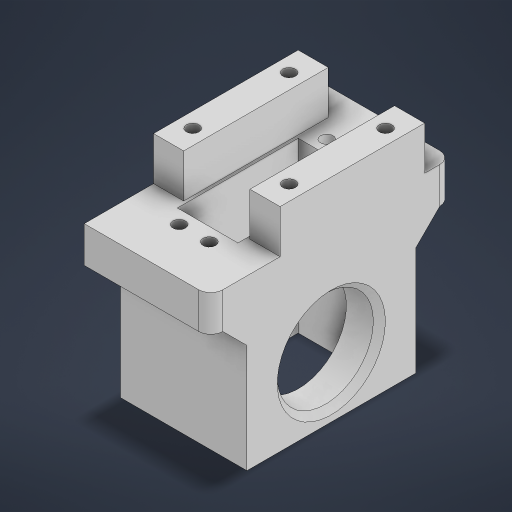
# Autodesk Inventor part: VerticalAxisServoMount
Saved by Autodesk Inventor 2024 (Build 280153000, 153)
## iProperties
Created: 2024-01-29
Part Number: VerticalAxisServoMount
Material: Generic
Document SubType Name: Modeling
Designer: avsar
Density: 1 g/cm^3
Appearance: Default
Author: avsar
Autodesk Inventor part; units mm, degrees
ref_plane "YZ Plane" through (0, 0, 0) normal (1, 0, 0) x (0, 1, 0)
ref_plane "XZ Plane" through (0, 0, 0) normal (0, 1, 0) x (-1, 0, 0)
ref_plane "XY Plane" through (0, 0, 0) normal (0, 0, 1) x (1, 0, 0)
sketch "Sketch1" plane through (0, 0, 0) normal (1, 0, 0) x (0, 1, 0)
  circle A0 centre (0, 0) radius 15.95
  dimension "d0" = 31.9
  constraints: 1 centre point, 1 coincident
  measures "d0" diameter of A0
extrude "Extrusion1" add sketch "Sketch1" along normal blind 8
sketch "Sketch2" plane through (8, 0, 0) normal (1, 0, 0) x (0, 0, -1)
  line L0 (-28, -20) -> (28, -20)
  line L1 (28, -20) -> (28, 36)
  line L2 (28, 36) -> (-28, 36)
  line L3 (-28, 36) -> (-28, -20)
  line L4 (-28, -20) -> (28, 36) construction
  line L5 (28, -20) -> (-28, 36) construction
  point P0 (0, 0)
  point P1 (0, 8)
  point P2 (0, 8)
  dimension "d3" = 56
  dimension "d4" = 56
  dimension "d46" = 8
  constraints: 12 end point, 2 midpoint, 2 parallel, 1 horizontal, 1 perpendicular, 1 vertical alignment
  measures "d3" distance of L1.end L0.end
  measures "d4" distance of L1.end L2.end
  measures "d46" distance of point (0, 0) point (0, 8)
extrude "Extrusion2" add sketch "Sketch2" along normal blind 42
sketch "Sketch3" plane through (8, 36, 28) normal (0, 1, 0) x (1, 0, 0)
  line L0 (0, 56) -> (42, 56) projected
  line L1 (21, 56) -> (21, 0) construction
  line L2 (0, 0) -> (42, 0) projected
  line L3 (10.95, 7.95) -> (31.05, 7.95)
  line L4 (31.05, 7.95) -> (31.05, 48.05)
  line L5 (31.05, 48.05) -> (10.95, 48.05)
  line L6 (10.95, 48.05) -> (10.95, 7.95)
  line L7 (10.95, 7.95) -> (31.05, 48.05) construction
  line L8 (31.05, 7.95) -> (10.95, 48.05) construction
  point P0 (-8, 28)
  point P1 (21, 28)
  dimension "d7" = 20.1
  dimension "d8" = 40.1
  constraints: 14 end point, 5 midpoint, 2 parallel, 1 horizontal, 1 perpendicular
  measures "d7" distance of L5.end L4.end
  measures "d8" distance of L4.end L3.end
extrude "Extrusion3" cut sketch "Sketch3" against normal through all
sketch "Sketch4" plane through (50, 0, 0) normal (1, 0, 0) x (0, 0, -1)
  circle A0 centre (0, 0) radius 15.95 projected
extrude "Extrusion4" cut sketch "Sketch4" against normal up to surface (10.95 mm away)
sketch "Sketch5" plane through (18.95, 36, 20.05) normal (1, 0, 0) x (0, 0, -1)
  circle A0 centre (20.05, -36) radius 15.95 construction
  circle A1 centre (12.05, -28) radius 2.1
  circle A2 centre (12.05, -44) radius 2.1
  circle A3 centre (28.05, -44) radius 2.1
  circle A4 centre (28.05, -28) radius 2.1
  dimension "d13" = 4.2
  dimension "d14" = 8
  dimension "d15" = 8
  dimension "d18" = 360
  constraints: 4 centre point, 9 other
  measures "d13" diameter of A1
  measures "d14" horizontal distance of A1.centre point (20.05, -36)
  measures "d15" horizontal distance of point (20.05, -36) A1.centre
extrude "Extrusion5" cut sketch "Sketch5" against normal through all
sketch "Sketch6" plane through (8, 36, 28) normal (0, 1, 0) x (1, 0, 0)
  line L0 (31.05, 48.05) -> (10.95, 48.05) construction
  line L1 (21, 48.05) -> (21, 7.95) construction
  line L2 (10.95, 7.95) -> (31.05, 7.95) construction
  line L3 (0, 0) -> (42, 0) projected
  line L4 (0, 0) -> (42, 0)
  line L5 (42, 0) -> (42, -12)
  line L6 (42, -12) -> (0, -12)
  line L7 (0, -12) -> (0, 0)
  line L8 (10.95, 7.95) -> (10.95, 48.05) construction
  line L9 (10.95, 28) -> (31.05, 28) construction
  line L10 (31.05, 12.05) -> (31.05, 43.95) construction
  line L11 (0, 56) -> (42, 56)
  line L12 (0, 56) -> (42, 56)
  line L13 (42, 56) -> (42, 68)
  line L14 (42, 68) -> (0, 68)
  line L15 (0, 68) -> (0, 56)
  point P0 (-8, 28)
  point P1 (21, 28)
  dimension "d25" = 12
  constraints: 22 end point, 5 midpoint, 5 symmetric about line, 2 parallel, 1 coincident, 1 horizontal, 1 perpendicular
  measures "d25" distance of L4.end L5.end
extrude "Extrusion6" add sketch "Sketch6" against normal blind 12
sketch "Sketch8" plane through (8, 36, 40) normal (0, 1, 0) x (1, 0, 0)
  line L0 (10.95, 19.95) -> (31.05, 19.95) construction
  line L1 (21, 19.95) -> (21, 60.05) construction
  line L2 (31.05, 60.05) -> (10.95, 60.05) construction
  circle A0 centre (26, 15.5) radius 2.1
  line L3 (31.05, 19.95) -> (10.95, 19.95) projected
  line L4 (10.95, 19.95) -> (10.95, 60.05) construction
  line L5 (10.95, 40) -> (31.05, 40) construction
  line L6 (31.05, 24.05) -> (31.05, 55.95) construction
  circle A1 centre (16, 15.5) radius 2.1
  circle A2 centre (26, 64.5) radius 2.1
  circle A3 centre (16, 64.5) radius 2.1
  point P0 (-8, 40)
  point P1 (21, 19.95)
  point P2 (21, 40)
  dimension "d31" = 4.2
  dimension "d32" = 5
  dimension "d33" = 24.5
  constraints: 6 midpoint, 4 centre point, 4 end point, 3 symmetric about line, 3 other
  measures "d31" diameter of A0
  measures "d32" horizontal distance of point (21, 19.95) A0.centre
  measures "d33" vertical distance of point (21, 40) A0.centre
extrude "Extrusion8" cut sketch "Sketch8" against normal up to surface (12 mm away)
fillet "Fillet2" radius 4 2 edges at (50, 30, 40) (50, 30, -40)
chamfer "Chamfer1" distance 2 angle 45 1 edges at (50, 0, 15.95)
chamfer "Chamfer2" distance 8 angle 45 2 edges at (29, 24, 28) (29, 24, -28)
sketch "Sketch10" plane through (8, 36, 40) normal (0, 1, 0) x (1, 0, 0)
  line L0 (31.05, 60.05) -> (10.95, 60.05) construction
  line L1 (21, 60.05) -> (21, 19.95) construction
  line L2 (31.05, 19.95) -> (10.95, 19.95) construction
  circle A0 centre (5, 31) radius 2.1
  circle A1 centre (5, 63) radius 2.1
  circle A2 centre (37, 31) radius 2.1
  circle A3 centre (37, 63) radius 2.1
  line L3 (0, 80) -> (0, 0) construction
  line L4 (0, 71) -> (10, 71)
  line L5 (10, 71) -> (10, 23)
  line L6 (10, 23) -> (0, 23)
  line L7 (0, 23) -> (0, 71)
  line L8 (5, 63) -> (5, 31) construction
  line L9 (42, 71) -> (32, 71)
  line L10 (32, 71) -> (32, 23)
  line L11 (32, 23) -> (42, 23)
  line L12 (42, 23) -> (42, 71)
  point P0 (-8, 40)
  point P1 (21, 40)
  point P2 (10, 47)
  point P3 (5, 47)
  dimension "d58" = 4.2
  dimension "d59" = 9
  dimension "d60" = 16
  dimension "d61" = 4.2
  dimension "d62" = 32
  dimension "d63" = 48
  dimension "d64" = 10
  constraints: 20 end point, 6 symmetric about line, 5 midpoint, 4 centre point, 2 parallel, 1 horizontal, 1 horizontal alignment, 1 perpendicular, 1 point on line, 1 vertical, 1 vertical alignment, 2 other
  measures "d58" diameter of A0
  measures "d59" vertical distance of point (21, 40) L8.end
  measures "d60" horizontal distance of point (21, 40) L8.end
  measures "d61" diameter of A1
  measures "d62" distance of L8.end L8.start
  measures "d63" distance of L4.end L5.end
  measures "d64" distance of L4.start L4.end
extrude "Extrusion10" add sketch "Sketch10" along normal blind 14.4
body "Solid1"
